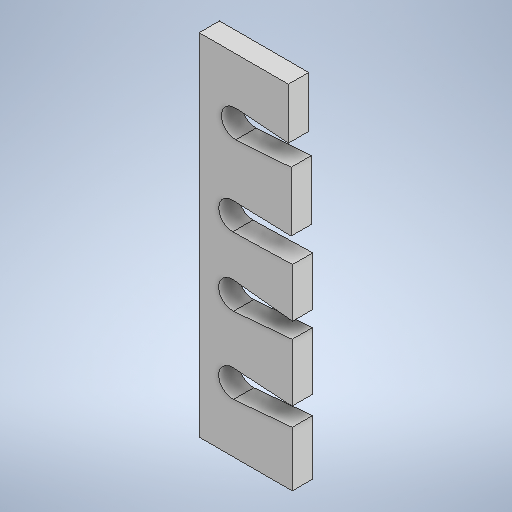
# Autodesk Inventor part: Part4
Saved by Autodesk Inventor 2025.3 (Build 293356000, 356)
## iProperties
Created: 2025-07-04
Part Number: Part4
Material: Generic
Document SubType Name: Modeling
Designer: steve
Density: 1 g/cm^3
Appearance: Default
Author: steve
Autodesk Inventor part; units mm, degrees
ref_plane "YZ Plane" through (0, 0, 0) normal (1, 0, 0) x (0, 1, 0)
ref_plane "XZ Plane" through (0, 0, 0) normal (0, 1, 0) x (-1, 0, 0)
ref_plane "XY Plane" through (0, 0, 0) normal (0, 0, 1) x (1, 0, 0)
sketch "Sketch1" plane through (0, 0, 0) normal (0, 0, 1) x (1, 0, 0)
  line L0 (0, 0) -> (0, 51.75)
  line L1 (0, 51.75) -> (13.18, 51.75)
  line L2 (13.18, 51.75) -> (13.18, 52.96)
  line L3 (13.18, 52.96) -> (0, 51.75)
  line L4 (13.18, 52.96) -> (13.18, 44.21)
  line L5 (13.58, 41.3175) -> (13.58, 32.5175)
  line L6 (13.79, 28.9779) -> (13.79, 21.7279)
  line L7 (13.74, 19.3888) -> (13.74, 10.8488)
  line L8 (13.75, 8.13) -> (13.75, 0)
  line L9 (0, 0) -> (13.75, 0)
  arc A0 (5.0261, 11.3943) -> (5.0771, 7.3661) centre (4.8999, 9.3783) ccw
  arc A1 (5.1161, 22.6617) -> (5.0736, 18.6408) centre (4.8999, 20.6533) ccw
  arc A2 (4.9633, 32.7882) -> (4.952, 28.7499) centre (4.8999, 30.7692) ccw
  arc A3 (5.4426, 44.7961) -> (5.4262, 40.7665) centre (5.29, 42.7819) ccw
  line L10 (13.18, 44.21) -> (5.4426, 44.7961)
  line L11 (13.58, 41.3175) -> (5.4262, 40.7665)
  line L12 (13.58, 32.5175) -> (4.9633, 32.7882)
  line L13 (13.79, 28.9779) -> (4.952, 28.7499)
  line L14 (13.79, 21.7279) -> (5.1161, 22.6617)
  line L15 (13.74, 19.3888) -> (5.0736, 18.6408)
  line L16 (13.74, 10.8488) -> (5.0261, 11.3943)
  line L17 (13.75, 8.13) -> (5.0771, 7.3661)
  point P0 (13.58, 36.9175)
  point P1 (0, 25.875)
  point P2 (13.79, 25.3529)
  point P3 (13.75, 4.065)
  dimension "d0" = 51.75
  dimension "d1" = 13.18
  dimension "d2" = 1.21
  dimension "d3" = 8.75
  dimension "d5" = 8.8
  dimension "d6" = 13.58
  dimension "d7" = 7.25
  dimension "d8" = 13.79
  dimension "d9" = 8.54
  dimension "d10" = 13.74
  dimension "d11" = 8.13
  dimension "d12" = 13.75
  dimension "d13" = 4.04
  dimension "d14" = 4.04
  dimension "d15" = 4.04
  dimension "d16" = 4.04
  dimension "d17" = 7.89
  constraints: 36 end point, 8 point on circle, 8 tangent, 6 vertical, 4 centre point, 4 midpoint, 2 perpendicular, 1 horizontal
  measures "d0" distance of L0.start L0.end
  measures "d1" distance of L0.end L1.end
  measures "d2" distance of L1.end L2.end
  measures "d3" distance of L2.end L4.end
  measures "d5" distance of L5.start L5.end
  measures "d6" distance from line of L0 point (13.58, 36.918)
  measures "d7" distance of L6.start L6.end
  measures "d8" horizontal distance of point (0, 25.875) point (13.79, 25.353)
  measures "d9" distance of L7.start L7.end
  measures "d10" distance between parallel lines of L0 L7
  measures "d11" distance of L8.start L8.end
  measures "d12" distance from line of L0 point (13.75, 4.065)
  measures "d13" diameter of A0
  measures "d14" diameter of A1
  measures "d15" diameter of A2
  measures "d16" diameter of A3
  measures "d17" distance from line of L4 A3.centre
extrude "Extrusion1" add sketch "Sketch1" along normal blind 3 contours L0 L1 L4 L10 A3 L11 L5 L12 A2 L13 L6 L14 A1 L15 L7 L16 A0 L17 L8 L9
body "Solid1"
